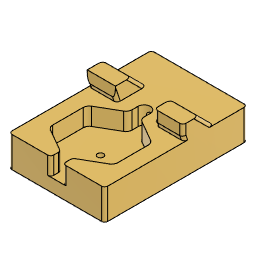
DiskDrillJig_Parametric (Autodesk Fusion 360 design; units mm, degrees)
Autodesk Fusion 360 part; units mm, degrees
note: some values were not read from the file. Chosen so that the rebuilt part matches the saved one: which face or edge a step refers to; which pieces of a blend or face edit are solid. Set by a fixed rule: which sketch regions a step uses.
sketch "Sketch1" plane through (0, 0, 0) normal (0, 0, 1) x (1, 0, 0)
  line L0 (15.65, 23.2976) -> (-15.65, 23.2976)
  line L1 (-15.65, 23.2976) -> (-15.65, -23.2976)
  line L2 (-15.65, -23.2976) -> (15.65, -23.2976)
  line L3 (15.65, -23.2976) -> (15.65, 23.2976)
  line L4 (15.65, 23.2976) -> (-15.65, -23.2976) construction
  line L5 (-15.65, 23.2976) -> (15.65, -23.2976) construction
  dimension "d1" = 46.5951
  dimension "d2" = 31.3
  constraint horizontal L0
  constraint perpendicular L0 L1
  constraint parallel L0 L2
  constraint parallel L1 L3
  constraint coincident L4 origin
  constraint coincident L5 origin
  measures "d1" distance of L0.end L1.end
  measures "d2" distance of L1.end L2.end
extrude "Extrude1" add sketch "Sketch1" along normal blind 10
sketch "Sketch2" plane through (0, 0, 10) normal (0, 0, 1) x (-1, 0, 0)
  line L0 (-15.65, 23.2976) -> (-15.65, -23.2976)
  line L1 (-15.65, -23.2976) -> (15.65, -23.2976)
  line L2 (15.65, -23.2976) -> (15.65, 23.2976)
  line L3 (15.65, 23.2976) -> (-15.65, 23.2976)
  line L4 (0, -3.2976) -> (15.65, 5.738)
  line L5 (15.65, 5.738) -> (15.65, 23.2976)
  line L6 (15.65, 23.2976) -> (-15.65, 23.2976)
  line L7 (-15.65, 23.2976) -> (-15.65, 5.738)
  line L8 (-15.65, 5.738) -> (0, -3.2976)
  line L9 (0, -3.2976) -> (0, 23.2976) construction
  line L10 (0, -3.2976) -> (10.65, 2.8512)
  line L11 (10.65, 2.8512) -> (10.65, 15.1488)
  line L12 (10.65, 15.1488) -> (0, 21.2976)
  line L13 (0, 21.2976) -> (-10.65, 15.1488)
  line L14 (-10.65, 15.1488) -> (-10.65, 2.8512)
  line L15 (-10.65, 2.8512) -> (0, -3.2976)
  point P0 (0, 9)
  dimension "d5" = 120
  dimension "d6" = 20
  dimension "d51" = 21.3
  constraint parallel L0 L5
  constraint perpendicular L0 L6
  constraint perpendicular L6 L7
  constraint horizontal L4.end L7.end
  constraint midpoint L6 L9.end
  constraint vertical L9
  constraint vertical origin L9.end
  constraint coincident L0.start L3.end
  constraint coincident L9 P0
  constraint vertical L14
  measures "d5" angle of L4 L8
  measures "d6" distance of L1 L4.start
  measures "d51" distance of L11 L14
extrude "Extrude2" cut sketch "Sketch2" against normal blind 5.75 contours L4 L8 L10 L11 L12 L13 L14 L15
sketch "Sketch3" plane through (0, 23.2976, 0) normal (0, 1, 0) x (-1, 0, 0)
  line L0 (-15.65, 0) -> (15.65, 0)
  line L1 (15.65, 0) -> (15.65, 10)
  line L2 (15.65, 10) -> (-15.65, 10)
  line L3 (-15.65, 10) -> (-15.65, 0)
  circle A0 centre (0, 7.25) radius 1
  line L4 (-10.65, 4.25) -> (0, 4.25)
  dimension "d10" = 2
  dimension "d60" = 3
  measures "d10" diameter of A0
  measures "d60" distance of A0.centre L4
extrude "Extrude3" cut sketch "Sketch3" against normal blind 34 contours A0
sketch "Sketch12" plane through (0, 0, 4.25) normal (0, 0, 1) x (-1, 0, 0)
  line L0 (-10.65, 2.8512) -> (0, -3.2976)
  line L1 (0, -3.2976) -> (10.65, 2.8512)
  line L2 (10.65, 2.8512) -> (10.65, 15.1488)
  line L3 (10.65, 15.1488) -> (0, 21.2976)
  line L4 (0, 21.2976) -> (-10.65, 15.1488)
  line L5 (-10.65, 15.1488) -> (-10.65, 2.8512)
  line L6 (0, -3.2976) -> (0, 21.2976) construction
  circle A0 centre (0, 9) radius 1
  dimension "d54" = 2
  constraint coincident L0.end L1.start
  constraint coincident L3.end L4.start
  constraint midpoint L6 A0.centre
  measures "d54" diameter of A0
extrude "Extrude10" cut sketch "Sketch12" against normal blind 9 contours A0
fillet "Fillet2" radius 2 4 edges at (10.65, -2.8512, 7.125) (10.65, -15.1488, 7.125) (-10.65, -2.8512, 7.125) (-10.65, -15.1488, 7.125)
sketch "Sketch5" plane through (0, 0, 10) normal (0, 0, 1) x (-1, 0, 0)
  line L0 (-15.65, -23.2976) -> (15.65, -23.2976)
  line L1 (15.65, -23.2976) -> (15.65, 23.2976)
  line L2 (9.65, 2.2739) -> (0, -3.2976)
  line L3 (0, -3.2976) -> (-9.65, 2.2739)
  line L4 (-15.65, 23.2976) -> (-15.65, -23.2976)
  line L5 (-2, 23.2976) -> (-2, -5.2976)
  arc A0 (-2, -5.2976) -> (2, -5.2976) centre (0, -5.2976) ccw
  line L6 (2, -5.2976) -> (2, 23.2976)
  arc A1 (2, 23.2976) -> (-2, 23.2976) centre (0, 23.2976) ccw
  line L7 (0, 23.2976) -> (0, -5.2976) construction
  line L8 (-10.65, 4.0059) -> (-10.65, 13.9941)
  line L9 (-9.65, 15.7261) -> (0, 21.2976)
  line L10 (0, 21.2976) -> (9.65, 15.7261)
  line L11 (10.65, 13.9941) -> (10.65, 4.0059)
  arc A2 (-10.65, 4.0059) -> (-9.65, 2.2739) centre (-8.65, 4.0059) ccw
  arc A3 (-9.65, 15.7261) -> (-10.65, 13.9941) centre (-8.65, 13.9941) ccw
  arc A4 (10.65, 13.9941) -> (9.65, 15.7261) centre (8.65, 13.9941) ccw
  arc A5 (9.65, 2.2739) -> (10.65, 4.0059) centre (8.65, 4.0059) ccw
  line L12 (15.65, 23.2976) -> (-15.65, 23.2976)
  line L13 (0, -3.2976) -> (0, -5.2976) construction
  dimension "d22" = 2
  dimension "d66" = 2
  constraint tangent L5 A0
  constraint tangent A0 L6
  constraint parallel L5 L6
  constraint tangent L6 A1
  constraint tangent L5 A1
  constraint vertical L7
  constraint vertical origin A1.centre
  constraint coincident A1.centre L12
  constraint coincident L2.end L3.start
  constraint coincident A0.centre L7.end
  measures "d22" radius of A0
  measures "d66" distance of L2.end A0.centre
extrude "Extrude5" cut sketch "Sketch5" against normal up to surface (5.75 mm away) contours L5 L6 L9 L10 L12 | A1 L12 | L2 L3 L5 L6 L9 L10 | L2 L3 L5 A0 L6
fillet "Fillet4" radius 2 2 edges at (-2, 2.1429, 7.125) (2, 2.1429, 7.125)
sketch "Sketch6" plane through (0, 0, 10) normal (0, 0, 1) x (-1, 0, 0)
  line L0 (-3, -1.5655) -> (-9.65, 2.2739)
  line L1 (-15.65, 23.2976) -> (-15.65, -23.2976)
  line L2 (-15.65, -23.2976) -> (15.65, -23.2976)
  line L3 (15.65, -23.2976) -> (15.65, 23.2976)
  line L4 (9.65, 2.2739) -> (3, -1.5655)
  line L5 (15.65, -7.2976) -> (-15.65, -7.2976)
  line L6 (-15.65, -7.2976) -> (-15.65, -2.2976)
  line L7 (-15.65, -2.2976) -> (15.65, -2.2976)
  line L8 (15.65, -2.2976) -> (15.65, -7.2976)
  line L9 (-10.65, 4.0059) -> (-10.65, 13.9941)
  line L10 (-9.65, 15.7261) -> (-2, 20.1429)
  line L11 (2, 20.1429) -> (9.65, 15.7261)
  line L12 (10.65, 13.9941) -> (10.65, 4.0059)
  arc A0 (-10.65, 4.0059) -> (-9.65, 2.2739) centre (-8.65, 4.0059) ccw
  arc A1 (-9.65, 15.7261) -> (-10.65, 13.9941) centre (-8.65, 13.9941) ccw
  arc A2 (10.65, 13.9941) -> (9.65, 15.7261) centre (8.65, 13.9941) ccw
  arc A3 (9.65, 2.2739) -> (10.65, 4.0059) centre (8.65, 4.0059) ccw
  line L13 (-2, 23.2976) -> (-15.65, 23.2976)
  arc A4 (-2, -3.2976) -> (-3, -1.5655) centre (-4, -3.2976) ccw
  arc A5 (3, -1.5655) -> (2, -3.2976) centre (4, -3.2976) ccw
  line L14 (2, 23.2976) -> (2, 20.1429)
  arc A6 (-2, -5.2976) -> (2, -5.2976) centre (0, -5.2976) ccw
  line L15 (-2, 20.1429) -> (-2, 23.2976)
  line L16 (2, -3.2976) -> (2, -5.2976)
  line L17 (15.65, 23.2976) -> (2, 23.2976)
  line L18 (-2, -5.2976) -> (-2, -3.2976)
  dimension "d28" = 5
  constraint horizontal L5
  constraint vertical L6
  constraint horizontal L7
  constraint vertical L8
  constraint coincident L1 L6.end
  constraint coincident L3 L5.start
  constraint tangent L5 A6
  measures "d28" distance of L5.end L6.end
extrude "Extrude6" add sketch "Sketch6" along normal blind 5 contours L1 L5 L6 L7 A4 A6 L18 | L7 A4 A5 A6 L16 L18 | L3 L5 L7 L8 A5 A6 L16
sketch "Sketch8" plane through (15.65, 0, 0) normal (1, 0, 0) x (0, 1, 0)
  line L0 (23.2976, 10) -> (7.2976, 10)
  line L1 (7.2976, 15) -> (2.2976, 15)
  line L2 (2.2976, 15) -> (2.2976, 10)
  line L3 (-23.2976, 0) -> (23.2976, 0)
  line L4 (2.2976, 10) -> (2.7976, 10)
  line L5 (2.7976, 10) -> (2.2976, 11.5)
  line L6 (7.2976, 10) -> (7.2976, 15)
  line L7 (23.2976, 0) -> (23.2976, 10)
  line L8 (2.2976, 10) -> (-23.2976, 10)
  line L9 (-23.2976, 10) -> (-23.2976, 0)
  dimension "d57" = 1.5
  dimension "d58" = 0.5
  constraint coincident L2.end L4.start
  constraint perpendicular L2 L4
  constraint coincident L2 L5.end
  measures "d57" distance of L2.end L5.end
  measures "d58" distance of L2.end L4.end
extrude "Extrude9" cut sketch "Sketch8" against normal through all contours L2 L4 L5
sketch "Sketch9" plane through (0, 0, 15) normal (0, 0, 1) x (-1, 0, 0)
  line L0 (15.65, -2.2976) -> (-15.65, -2.2976)
  line L1 (-15.65, -2.2976) -> (-15.65, -7.2976)
  line L2 (15.65, -7.2976) -> (15.65, -2.2976)
  line L3 (-6.39, -7.2976) -> (6.39, -7.2976)
  line L4 (6.39, -7.2976) -> (6.39, -2.2976)
  line L5 (6.39, -2.2976) -> (-6.39, -2.2976)
  line L6 (-6.39, -2.2976) -> (-6.39, -7.2976)
  line L7 (-6.39, -7.2976) -> (6.39, -2.2976) construction
  line L8 (6.39, -7.2976) -> (-6.39, -2.2976) construction
  line L9 (-15.65, -7.2976) -> (15.65, -7.2976)
  point P0 (0, -4.7976)
  dimension "d43" = 12.78
  constraint horizontal L3
  constraint perpendicular L3 L4
  constraint parallel L3 L5
  constraint parallel L4 L6
  constraint coincident L7 P0
  constraint coincident L8 P0
  constraint coincident L0 L5.end
  constraint vertical origin P0
  constraint coincident L3.start L9
  measures "d43" distance of L4.end L5.end
extrude "Extrude8" cut sketch "Sketch9" against normal blind 5 contours L0 L3 L4 L5 L6 L9
chamfer "Chamfer1" distance 5 angle 45 2 edges at (7.825, 7.2976, 10) (-7.825, 7.2976, 10)
fillet "Fillet6" radius 1 10 edges at (15.65, 2.2976, 13.25) (15.65, 9.7976, 12.5) (-15.65, 9.7976, 12.5) (6.39, 2.2976, 13.25) (6.39, 9.7976, 12.5) (-6.39, 9.7976, 12.5) (15.65, 2.5476, 10.75) (6.39, 2.5476, 10.75) (-6.39, 2.5476, 10.75) (-15.65, 2.5476, 10.75)
fillet "Fillet3" radius 1 4 edges at (-15.65, -23.2976, 5) (15.65, -23.2976, 5) (-15.65, 23.2976, 5) (15.65, 23.2976, 5)
fillet "Fillet7" radius 1 4 edges at (2, -20.1429, 7.125) (2, -23.2976, 7.125) (-2, -23.2976, 7.125) (-2, -20.1429, 7.125)
equation "d1 = D / 0.86602540378 + 22 mm"
equation "d2 = D + 10 mm"
equation "d3 = h + 4 mm"
equation "d7 = -( h - 0.25 mm )"
equation "d43 = D * 0.6"
equation "d51 = D"
equation "D = 21.3 mm" comment "Pad Diameter"
equation "h = 6 mm" comment "Pad Height"
named bodies: "DiskDrillRig_3mm"
